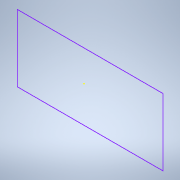
# Autodesk Inventor part: spoil board
Saved by Autodesk Inventor 2020.2 (Build 242310000, 310)
## iProperties
Created: 2020-04-02
Part Number: spoil board
Material: Generic
Document SubType Name: Modeling
Designer: deli
Density: 1 g/cm^3
Appearance: Default
Author: deli
Autodesk Inventor part; units mm, degrees
ref_plane "YZ Plane" through (0, 0, 0) normal (1, 0, 0) x (0, 1, 0)
ref_plane "XZ Plane" through (0, 0, 0) normal (0, 1, 0) x (-1, 0, 0)
ref_plane "XY Plane" through (0, 0, 0) normal (0, 0, 1) x (1, 0, 0)
sketch "Sketch1" plane through (0, 0, 0) normal (0, 0, 1) x (1, 0, 0)
  line L0 (-1218.5157, 565.8874) -> (1219.8843, 565.8874)
  line L1 (1219.8843, 565.8874) -> (1219.8843, -653.3126)
  line L2 (1219.8843, -653.3126) -> (-1218.5157, -653.3126)
  line L3 (-1218.5157, -653.3126) -> (-1218.5157, 565.8874)
  point P0 (0, 0)
  dimension "d2" = 1219.2
  dimension "d3" = 2438.4
  constraints: 8 end point, 2 parallel, 1 horizontal, 1 perpendicular
  measures "d2" distance of L2.end L0.start
  measures "d3" distance of L0.start L0.end
extrude "Extrusion1" add sketch "Sketch1" along normal blind 19.05
body "Solid1"
